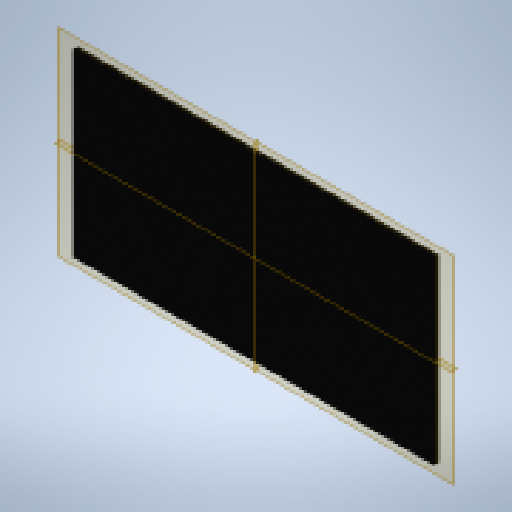
# Autodesk Inventor part: Peça9_mesa
Saved by Autodesk Inventor 2025.2 (Build 292293000, 293)
## iProperties
Created: 2025-03-28
Part Number: Peça9_mesa
Material: Aço galvanizado
Document SubType Name: Sheet Metal
Designer: Formação
Density: 7.85 g/cm^3
Sheet Metal Rule: Padrão_mm
Appearance: Preto
Author: Formação
Autodesk Inventor part; units mm, degrees
sketch "Esboço1" plane through (0, 0, 0) normal (0, 0, 1) x (1, 0, 0)
  line L0 (-750, 375) -> (750, 375)
  line L1 (750, 375) -> (750, -375)
  line L2 (750, -375) -> (-750, -375)
  line L3 (-750, -375) -> (-750, 375)
  line L4 (-750, 375) -> (750, -375) construction
  line L5 (750, 375) -> (-750, -375) construction
  point P0 (0, 0)
  point P1 (0, 0)
  dimension "d0" = 1500
  dimension "d1" = 750
  constraints: 12 end point, 2 midpoint, 2 parallel, 1 coincident, 1 horizontal, 1 perpendicular
  measures "d0" distance of L1.end L2.end
  measures "d1" distance of L1.end L0.end
extrude "Extrusão1" add sketch "Esboço1" along normal mid plane 20
sketch "Esboço2" plane through (0, 0, 10) normal (0, 0, 1) x (1, 0, 0)
  circle A0 centre (-650, 300) radius 9.5
  circle A1 centre (-650, 300) radius 11.5
  point P0 (0, 0)
  dimension "d4" = 19
  dimension "d5" = 650
  dimension "d6" = 300
  dimension "d11" = 23
  dimension "d12" = 2
  constraints: 2 centre point, 1 concentric
  measures "d4" diameter of A0
  measures "d5" horizontal distance of point (0, 0) A0.centre
  measures "d6" vertical distance of point (0, 0) A0.centre
  measures "d11" diameter of A1
  measures "d12" radial gap between concentric circles of A1 A0
extrude "Extrusão3" cut sketch "Esboço2" against normal blind 10
mirror "Espelhar3" about plane through (0, 0, 0) normal (1, 0, 0) of "Extrusão3"
mirror "Espelhar4" about plane through (0, 0, 0) normal (0, 1, 0) of "Extrusão3", "Espelhar3"
fillet "Arredondamento1" radius 5 1 edges at (-750, 375, 0)
mirror "Espelhar5" about plane through (0, 0, 0) normal (1, 0, 0) of "Arredondamento1"
mirror "Espelhar6" about plane through (0, 0, 0) normal (0, 1, 0) of "Arredondamento1", "Espelhar5"
equation "\"Raio_vergadura\" = Espessura"
equation "\"Largura_alívio_de_vergadura\" = Espessura"
equation "\"Profundidade_alívio_de_vergadura\" = 0.5 * Espessura"
equation "\"Tamanho_alívio_de_dobra\" = 4 * Espessura"
equation "\"Remanescente_mínimo\" = 2 * Espessura"
equation "\"Raiodetransição\" = Raio_vergadura"
equation "\"Tamanho_de_raio_de_Jacobi\" = Raio_vergadura"
equation "\"TamanhoFolga\" = Espessura"
equation "\"Espessura\" = 0.5"
